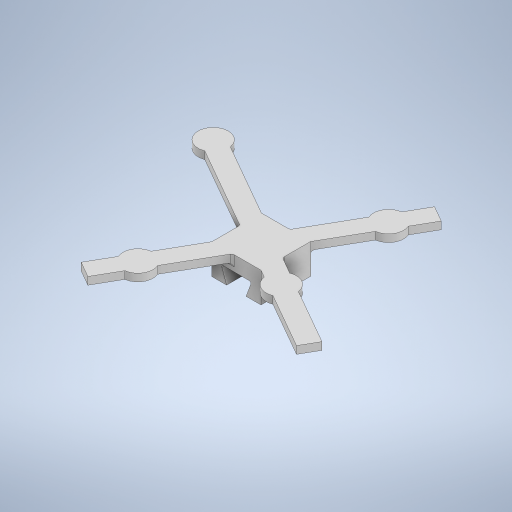
# Autodesk Inventor part: female1
Saved by Autodesk Inventor 2023 (Build 270158000, 158)
## iProperties
Created: 2024-01-15
Part Number: female1
Material: Generic
Document SubType Name: Modeling
Designer: User
Density: 1 g/cm^3
Appearance: Default
Author: User
Autodesk Inventor part; units mm, degrees
ref_plane "YZ Plane" through (0, 0, 0) normal (1, 0, 0) x (0, 1, 0)
ref_plane "XZ Plane" through (0, 0, 0) normal (0, 1, 0) x (-1, 0, 0)
ref_plane "XY Plane" through (0, 0, 0) normal (0, 0, 1) x (1, 0, 0)
sketch "Sketch1" plane through (0, 0, 0) normal (0, 0, 1) x (1, 0, 0)
  line L0 (0, 5) -> (4.285926, 5)
  line L1 (4.755772, 4.32899) -> (3.180149, 0)
  line L2 (3.180149, 0) -> (0, 0)
  line L3 (0, 5) -> (-4.285926, 5)
  line L4 (-4.755772, 4.32899) -> (-3.180149, 0)
  line L5 (-3.180149, 0) -> (0, 0)
  arc A0 (-4.285926, 5) -> (-4.755772, 4.32899) centre (-4.285926, 4.5) ccw
  arc A1 (4.755772, 4.32899) -> (4.285926, 5) centre (4.285926, 4.5) ccw
  line L6 (4.285926, 5.05) -> (0, 5.05)
  line L7 (0, 5.05) -> (-4.285926, 5.05)
  arc A2 (-4.285926, 5.05) -> (-4.802757, 4.311889) centre (-4.285926, 4.5) ccw
  line L8 (-4.802757, 4.311889) -> (-3.215159, -0.05)
  line L9 (-3.215159, -0.05) -> (0, -0.05)
  line L10 (0, -0.05) -> (3.215159, -0.05)
  line L11 (3.215159, -0.05) -> (4.802757, 4.311889)
  arc A3 (4.802757, 4.311889) -> (4.285926, 5.05) centre (4.285926, 4.5) ccw
  line L12 (-3.180149, 0) -> (-8.180149, 0)
  line L13 (-8.180149, 0) -> (-8.180149, 7.5)
  line L14 (3.180149, 0) -> (8.180149, 0)
  line L15 (8.180149, 0) -> (8.180149, 7.5)
  line L16 (8.180149, 7.5) -> (-8.180149, 7.5)
  point P0 (5, 5)
  point P1 (-5, 5)
  point P2 (3.233358, 0)
  point P3 (-3.233358, 0)
  dimension "d0" = 5
  dimension "d1" = 5
  dimension "d2" = 70
  dimension "d3" = 5
  dimension "d4" = 70
  dimension "d5" = 0.5
  dimension "d6" = 0.05
  dimension "d7" = 5
  dimension "d8" = 7.5
  dimension "d9" = 5
  constraints: 34 end point, 8 point on circle, 7 point on line, 4 centre point, 4 parallel, 4 tangent, 3 perpendicular, 1 equal radius, 1 horizontal, 7 other
  measures "d0" distance of L2.end L0.start
  measures "d1" distance of L0.start point (5, 5)
  measures "d2" angle of L0 L1
  measures "d3" distance of L0.start point (-5, 5)
  measures "d4" angle of L4 L3
  measures "d5" radius of A0
  measures "d6" distance between parallel lines of L0 L6
  measures "d7" distance of L4.end L12.end
  measures "d8" distance of L12.end L13.end
  measures "d9" distance of L1.end L14.end
extrude "Extrusion1" add sketch "Sketch1" along normal blind 16.5 contours L11 A3 L6 L7 A2 L8 L12 L13 L16 L15 L14
sketch "Sketch2" plane through (-8.180149, 7.5, 0) normal (0, 1, 0) x (1, 0, 0)
  line L0 (-10.580957, -47.057485) -> (32.148268, 27.576377)
  line L1 (32.148268, 27.576377) -> (26.941254, 30.557485)
  line L2 (26.941254, 30.557485) -> (-15.78797, -44.076377)
  line L3 (-15.78797, -44.076377) -> (-10.580957, -47.057485)
  line L4 (-10.580957, -47.057485) -> (26.941254, 30.557485) construction
  line L5 (32.148268, 27.576377) -> (-15.78797, -44.076377) construction
  circle A0 centre (-6.725395, -34.285068) radius 5
  circle A1 centre (23.582544, 18.652904) radius 5
  line L6 (-13.184463, -45.566931) -> (29.544761, 29.066931) construction
  line L7 (16.360298, -16.5) -> (0, -16.5) construction
  line L8 (0, 0) -> (16.360298, -16.5) construction
  line L9 (16.360298, 0) -> (0, 0) construction
  line L10 (16.360298, -16.5) -> (16.360298, 0) construction
  line L11 (16.360298, 0) -> (0.368439, -15.856459) construction
  line L12 (-30.674699, 10.428379) -> (-27.598866, 15.800845)
  line L13 (-27.598866, 15.800845) -> (47.034997, -26.928379)
  line L14 (47.034997, -26.928379) -> (43.959163, -32.300845)
  line L15 (43.959163, -32.300845) -> (-30.674699, 10.428379)
  line L16 (-30.674699, 10.428379) -> (47.034997, -26.928379) construction
  line L17 (-27.598866, 15.800845) -> (43.959163, -32.300845) construction
  circle A2 centre (-29.136782, 13.114612) radius 5
  circle A3 centre (23.80119, -17.193326) radius 5
  line L18 (-29.136782, 13.114612) -> (45.49708, -29.614612)
  point P0 (8.180149, 0)
  point P1 (8.180149, -8.25)
  point P2 (8.180149, -8.25)
  point P3 (-24.191137, 13.849859)
  point P4 (-27.26697, 8.477393)
  point P5 (4.038725, -9.445679)
  point P6 (-7.341496, -29.323171)
  point P7 (-11.316307, -36.265856)
  point P8 (-6.109293, -39.246965)
  point P9 (-2.134482, -32.30428)
  point P10 (9.245739, -12.426788)
  point P11 (18.855544, -17.928573)
  point P12 (25.671002, -21.830545)
  point P13 (28.746835, -16.458079)
  point P14 (21.931377, -12.556107)
  point P15 (12.321572, -7.054321)
  point P16 (24.198645, 13.691007)
  point P17 (28.173456, 20.633692)
  point P18 (22.966443, 23.614801)
  point P19 (18.991631, 16.672116)
  point P20 (7.114559, -4.073212)
  dimension "d12" = 86
  dimension "d13" = 6
  dimension "d14" = 10
  dimension "d15" = 10
  dimension "d16" = 61
  dimension "d17" = 12
  dimension "d19" = 86
  dimension "d20" = 10
  dimension "d21" = 10
  dimension "d22" = 61
  dimension "d26" = 90
  constraints: 34 end point, 10 midpoint, 6 point on line, 4 centre point, 4 parallel, 4 perpendicular
  measures "d12" distance of L2.end L1.end
  measures "d13" distance of L0.end L1.end
  measures "d14" diameter of A0
  measures "d15" diameter of A1
  measures "d16" distance of A1.centre A0.centre
  measures "d17" distance from line of L1 A1.centre
  measures "d19" distance of L12.end L13.end
  measures "d20" diameter of A2
  measures "d21" diameter of A3
  measures "d22" distance of A3.centre L18.start
  measures "d26" angle of L2 L15
extrude "Extrusion2" add sketch "Sketch2" along normal blind 2.5
sketch "Sketch3" plane through (-8.180149, 7.5, 0) normal (0, 1, 0) x (1, 0, 0)
  line L0 (0, -7.133436) -> (0, -16.5)
  line L1 (9.446546, 0) -> (0, 0)
  line L2 (16.360298, 0) -> (16.360298, -9.366564)
  line L3 (16.360298, -16.5) -> (6.913752, -16.5)
  line L4 (0, 0) -> (4.946791, 0)
  line L5 (0, 0) -> (16.360298, 0)
  line L6 (16.360298, 0) -> (16.360298, -16.5)
  line L7 (16.360298, -16.5) -> (0, -16.5)
  line L8 (0, -16.5) -> (0, 0)
  point P0 (8.180149, 0)
  point P1 (0, -16.418433)
  point P2 (16.360298, -0.081567)
  point P3 (0, -16.418433)
  point P4 (16.360298, -0.081567)
  constraints: 8 end point, 2 parallel, 1 horizontal, 1 perpendicular
extrude "Extrusion3" add sketch "Sketch3" along normal blind 2.5
fillet "Fillet1" radius 1 8 edges at (4.7233, 7.5, 0) (1.2664, 8.75, 0) (-8.1801, 7.5, 3.5667) (-8.1801, 8.75, 7.1334) (-4.7233, 7.5, 16.5) (-1.2664, 8.75, 16.5) (8.1801, 7.5, 12.9333) (8.1801, 8.75, 9.3666)
body "Solid1"
